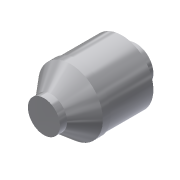
# Autodesk Inventor part: 00_Oxygen_Oxi
Saved by Autodesk Inventor 2019.4 (Build 234330000, 330)
## iProperties
Created: 2021-06-01
Part Number: 00_Oxygen_Oxi
Material: Generic
Document SubType Name: Modeling
Designer: diederichbenedict
Density: 1 g/cm^3
Appearance: Smooth - White
Author: diederichbenedict
Autodesk Inventor part; units mm, degrees
ref_plane "YZ Plane" through (0, 0, 0) normal (1, 0, 0) x (0, 1, 0)
ref_plane "XZ Plane" through (0, 0, 0) normal (0, 1, 0) x (-1, 0, 0)
ref_plane "XY Plane" through (0, 0, 0) normal (0, 0, 1) x (1, 0, 0)
sketch "Sketch1" plane through (0, 0, 0) normal (1, 0, 0) x (0, 1, 0)
  line L0 (0, 0) -> (7.78, 0)
  line L1 (7.78, 0) -> (7.78, 6.36)
  line L2 (7.78, 6.36) -> (14.1299, 6.36)
  line L3 (14.1299, 6.36) -> (14.1299, 25.9405)
  line L4 (14.1299, 25.9405) -> (14.5, 25.9405)
  line L5 (14.5, 25.9405) -> (14.5, 29.4359)
  line L6 (14.5, 29.4359) -> (7.21, 38.19)
  line L7 (7.21, 38.19) -> (7.21, 41.4)
  line L8 (7.21, 41.4) -> (0, 41.4)
  line L9 (0, 41.4) -> (0, 0)
  dimension "d0" = 7.78
  dimension "d1" = 6.36
  dimension "d2" = 41.4
  dimension "d3" = 7.21
  dimension "d4" = 14.5
  constraints: 20 end point, 7 perpendicular, 1 horizontal, 1 parallel
  measures "d0" distance of L0.start L0.end
  measures "d1" distance of L0.end L1.end
  measures "d2" distance between parallel lines of L0 L8
  measures "d3" distance between parallel lines of L9 L7
  measures "d4" distance from line of L9 L5.end
revolve "Revolution1" add sketch "Sketch1" angle 360 about axis through (0, 0, 41.4) along (0, 0, -1)
body "Solid1"
